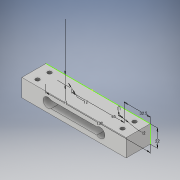
# Autodesk Inventor part: sc601_load_cell
Saved by Autodesk Inventor 2019 (Build 230136000, 136)
## iProperties
Created: 2019-02-09
Part Number: sc601_load_cell
Material: 一般
Document SubType Name: Modeling
Designer: drago
Density: 1 g/cm^3
Appearance: 既定
Author: drago
Autodesk Inventor part; units mm, degrees
ref_plane "YZ Plane" through (0, 0, 0) normal (1, 0, 0) x (0, 1, 0)
ref_plane "XZ Plane" through (0, 0, 0) normal (0, 1, 0) x (-1, 0, 0)
ref_plane "XY Plane" through (0, 0, 0) normal (0, 0, 1) x (1, 0, 0)
sketch "スケッチ1" plane through (0, 0, 0) normal (0, 0, 1) x (1, 0, 0)
  line L0 (-57.6728, -0.0614) -> (72.3272, -0.0614)
  line L1 (72.3272, -0.0614) -> (72.3272, -22.0614)
  line L2 (72.3272, -22.0614) -> (-57.6728, -22.0614)
  line L3 (-57.6728, -22.0614) -> (-57.6728, -0.0614)
  circle A0 centre (-25.1728, -11.0614) radius 6
  circle A1 centre (39.8272, -11.0614) radius 6
  line L4 (-21.2046, -6.5611) -> (35.8589, -6.5611)
  line L5 (-21.2046, -15.5617) -> (35.8589, -15.5617)
  point P0 (0, 0)
  dimension "d0" = 130
  dimension "d1" = 22
  dimension "d4" = 12
  dimension "d5" = 12
  dimension "d6" = 65
  dimension "d7" = 11
  dimension "d8" = 11
  dimension "d9" = 32.5
  constraints: 12 end point, 4 point on circle, 3 parallel, 2 centre point, 2 horizontal, 1 perpendicular
  measures "d0" distance of L1.end L2.end
  measures "d1" distance of L0.end L1.end
  measures "d4" diameter of A0
  measures "d5" diameter of A1
  measures "d6" distance of A1.centre A0.centre
  measures "d7" distance from line of L0 A1.centre
  measures "d8" distance from line of L0 A0.centre
  measures "d9" distance from line of L1 A1.centre
extrude "押し出し1" add sketch "スケッチ1" along normal blind 30 contours L0 L1 L2 L3 | A0 | A0 L4 A1 L5 | A1
extrude "押し出し2" cut sketch "スケッチ1" along normal blind 30 contours A0 | A0 L4 A1 L5 | A1
sketch "スケッチ2" plane through (-57.6728, -0.0614, 0) normal (0, 1, 0) x (1, 0, 0)
  circle A0 centre (12, -7.5) radius 3
  line L0 (65, -1.1982) -> (65, -25.359)
  line L1 (8.4096, -15) -> (24.5168, -15)
  line L2 (130, 0) -> (130, -30) projected
  line L3 (0, 0) -> (130, 0) projected
  line L4 (0, 0) -> (0, -30) projected
  circle A1 centre (12, -22.5) radius 3
  circle A2 centre (118, -7.5) radius 3
  circle A3 centre (118, -22.5) radius 3
  point P0 (57.6728, 0)
  dimension "d12" = 6
  dimension "d13" = 65
  dimension "d14" = 15
  dimension "d15" = 12
  dimension "d16" = 7.5
  constraints: 4 centre point, 4 end point, 3 symmetric about line, 1 horizontal, 1 vertical, 3 other
  measures "d12" diameter of A0
  measures "d13" distance between parallel lines of L2 L0
  measures "d14" distance between parallel lines of L3 L1
  measures "d15" distance from line of L4 A0.centre
  measures "d16" distance from line of L3 A0.centre
hole "穴1" at (-45.6728, -0.0614, 7.5) at (-45.6728, -0.0614, 22.5) at (60.3272, -0.0614, 7.5) at (60.3272, -0.0614, 22.5) direction (0, -1, 0) diameter 4.917 end through all thread size "M6x1" class "6H" standard "ANSI Metric M Profile"
